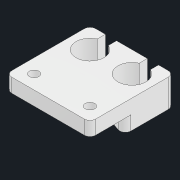
# Autodesk Inventor part: scara-base11
Saved by Autodesk Inventor 2022 (Build 260153000, 153)
## iProperties
Created: 2021-10-21
Part Number: scara-base11
Material: ABS プラスチック
Document SubType Name: Modeling
Designer: Yuta Kage
Density: 1.06 g/cm^3
Appearance: 滑らか - 白
Author: Yuta Kage
Autodesk Inventor part; units mm, degrees
ref_plane "YZ Plane" through (0, 0, 0) normal (1, 0, 0) x (0, 1, 0)
ref_plane "XZ Plane" through (0, 0, 0) normal (0, 1, 0) x (-1, 0, 0)
ref_plane "XY Plane" through (0, 0, 0) normal (0, 0, 1) x (1, 0, 0)
sketch "スケッチ1" plane through (0, 0, 0) normal (0, 1, 0) x (-1, 0, 0)
  line L0 (15, 10) -> (-15, 10)
  line L1 (-15, 10) -> (-15, -20)
  line L2 (-15, -20) -> (15, -20)
  line L3 (15, -20) -> (15, 10)
  line L4 (15, 10) -> (-15, -20) construction
  line L5 (-15, 10) -> (15, -20) construction
  point P0 (0, 0)
  point P1 (0, -5)
  dimension "d0" = 30
  dimension "d15" = 10
  dimension "d16" = 20
  constraints: 12 end point, 2 parallel, 1 horizontal, 1 midpoint, 1 perpendicular, 1 vertical alignment
  measures "d0" distance of L0.start L0.end
  measures "d15" distance from line of point (0, 0) L0
  measures "d16" distance from line of point (0, 0) L2
extrude "押し出し1" add sketch "スケッチ1" along normal mid plane 10
sketch "スケッチ2" plane through (0, 5, 0) normal (0, 1, 0) x (1, 0, 0)
  line L0 (-15, -10) -> (15, -10) projected
  point P0 (0, 0)
  point P1 (-10, -5)
  point P2 (10, -5)
  dimension "d4" = 10
  dimension "d5" = 10
  dimension "d6" = 5
  constraints: 1 horizontal alignment
  measures "d4" horizontal distance of point (0, 0) point (-10, -5)
  measures "d5" horizontal distance of point (0, 0) point (10, -5)
  measures "d6" distance from line of L0 point (-10, -5)
hole "穴1" at (-10, 5, 5) at (10, 5, 5) direction (0, -1, 0) diameter 3.4 end through all clearance for "Socket Head Cap Screw" size "M3" standard "Ansi Metric M Profile"
sketch "スケッチ3" plane through (0, -5, 0) normal (0, -1, 0) x (1, 0, 0)
  circle A0 centre (0, 30) radius 34.9965
  circle A1 centre (-10, 5) radius 1.7 projected
  point P0 (0, 0)
  dimension "d17" = 25
  dimension "d18" = 69.993
  constraints: 1 centre point, 1 vertical alignment
  measures "d17" vertical distance of A1.centre A0.centre
  measures "d18" diameter of A0
extrude "押し出し2" cut sketch "スケッチ3" against normal blind 5
fillet "フィレット1" radius 2 2 edges at (15, -2.5, -1.6189) (-15, -2.5, -1.6189)
fillet "フィレット2" radius 2 2 edges at (15, 2.5, 10) (-15, 2.5, 10)
fillet "フィレット3" radius 2 2 edges at (15, 0, -20) (-15, 0, -20)
sketch "スケッチ4" plane through (0, 5, 0) normal (0, 1, 0) x (1, 0, 0)
  circle A0 centre (-7.5, 12.5) radius 5
  circle A1 centre (7.5, 12.5) radius 5
  line L0 (13, 20) -> (-13, 20) projected
  line L1 (-15, 18) -> (-15, -8) projected
  line L2 (15, -8) -> (15, 18) projected
  point P0 (0, 0)
  dimension "d26" = 10
  dimension "d27" = 10
  dimension "d28" = 7.5
  dimension "d29" = 7.5
  dimension "d30" = 7.5
  dimension "d31" = 7.5
  constraints: 2 centre point
  measures "d26" diameter of A0
  measures "d27" diameter of A1
  measures "d28" distance from line of L0 A0.centre
  measures "d29" distance from line of L1 A0.centre
  measures "d30" distance from line of L0 A1.centre
  measures "d31" distance from line of L2 A1.centre
extrude "押し出し3" cut sketch "スケッチ4" against normal through all
sketch "スケッチ5" plane through (0, 5, 0) normal (0, 1, 0) x (1, 0, 0)
  circle A0 centre (-7.5, 12.5) radius 5 projected
  circle A1 centre (7.5, 12.5) radius 5 projected
  line L0 (-9.5, 17.0826) -> (-5.5, 17.0826)
  line L1 (-5.5, 17.0826) -> (-5.5, 20)
  line L2 (-5.5, 20) -> (-9.5, 20)
  line L3 (-9.5, 20) -> (-9.5, 17.0826)
  line L4 (-9.5, 17.0826) -> (-5.5, 20) construction
  line L5 (-5.5, 17.0826) -> (-9.5, 20) construction
  line L6 (5.5, 17.0826) -> (9.5, 17.0826)
  line L7 (9.5, 17.0826) -> (9.5, 20)
  line L8 (9.5, 20) -> (5.5, 20)
  line L9 (5.5, 20) -> (5.5, 17.0826)
  line L10 (5.5, 17.0826) -> (9.5, 20) construction
  line L11 (9.5, 17.0826) -> (5.5, 20) construction
  line L12 (13, 20) -> (-13, 20) projected
  point P0 (0, 0)
  point P1 (-7.5, 18.5413)
  point P2 (7.5, 18.5413)
  point P3 (-7.5, 18.5413)
  point P4 (7.5, 18.5413)
  dimension "d34" = 4
  dimension "d35" = 4
  constraints: 24 end point, 6 midpoint, 4 parallel, 2 horizontal, 2 perpendicular, 2 point on circle, 2 point on line, 2 vertical alignment, 2 other
  measures "d34" distance of L6.start L6.end
  measures "d35" distance of L0.start L0.end
extrude "押し出し4" cut sketch "スケッチ5" against normal through all contours L8 L7 A1 L9 | L0 A0 | A0 L3 L2 L1 | A1 L6 picked at (-7.8405, 17.1866) picked at (7.1595, 17.1866)
equation "\"d29\" = d28"
equation "\"d30\" = d28"
equation "\"d31\" = d29"
equation "\"d35\" = d34"
